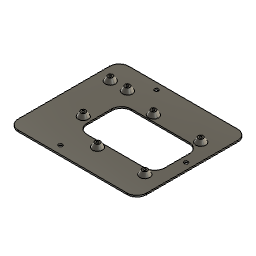
pi and feather sled (Autodesk Fusion 360 design; units mm, degrees)
Autodesk Fusion 360 part; units mm, degrees
sketch "Sketch1" plane through (0, 0, 0) normal (0, 0, 1) x (1, 0, 0)
  line L0 (0, 0) -> (203, 0) construction
  line L1 (203, 0) -> (203, 151) construction
  line L2 (203, 151) -> (0, 151) construction
  line L3 (0, 151) -> (0, 0) construction
  line L4 (101.5, 151) -> (101.5, 0) construction
  line L5 (0, 75.5) -> (203, 75.5) construction
  circle A0 centre (25.85, 110.5) radius 2
  circle A1 centre (61.05, 125.25) radius 2
  circle A2 centre (21, 75.5) radius 2
  circle A3 centre (101.5, 125.25) radius 2
  circle A4 centre (141.95, 125.25) radius 2
  circle A5 centre (177.15, 110.5) radius 2
  circle A6 centre (182, 75.5) radius 2
  circle A7 centre (25.85, 40.5) radius 2
  circle A8 centre (101.5, 25.75) radius 2
  circle A9 centre (61.05, 25.75) radius 2
  circle A10 centre (141.95, 25.75) radius 2
  circle A11 centre (177.15, 40.5) radius 2
  line L6 (122.4543, 101.192) -> (171.4543, 101.192) construction
  line L7 (171.4543, 101.192) -> (171.4543, 43.192) construction
  line L8 (171.4543, 43.192) -> (122.4543, 43.192) construction
  line L9 (122.4543, 43.192) -> (122.4543, 101.192) construction
  line L10 (118.9543, 124.692) -> (174.9543, 124.692) construction
  line L11 (174.9543, 124.692) -> (174.9543, 39.692) construction
  line L12 (174.9543, 39.692) -> (118.9543, 39.692) construction
  line L13 (118.9543, 39.692) -> (118.9543, 124.692) construction
  circle A12 centre (122.4543, 101.192) radius 1.15
  circle A13 centre (171.4543, 101.192) radius 1.15
  circle A14 centre (171.4543, 43.192) radius 1.15
  circle A15 centre (122.4543, 43.192) radius 1.15
  circle A16 centre (122.4543, 101.192) radius 2.65
  circle A17 centre (171.4543, 101.192) radius 2.65
  circle A18 centre (171.4543, 43.192) radius 2.65
  circle A19 centre (122.4543, 43.192) radius 2.65
  line L14 (55.9879, 132.0749) -> (188.973, 132.0749)
  line L15 (188.973, 132.0749) -> (188.973, 17.4198)
  line L16 (188.973, 17.4198) -> (55.9879, 17.4198)
  line L17 (55.9879, 17.4198) -> (55.9879, 132.0749)
  line L18 (69.6743, 109.192) -> (87.4543, 109.192) construction
  line L19 (87.4543, 109.192) -> (87.4543, 63.472) construction
  line L20 (87.4543, 63.472) -> (69.6743, 63.472) construction
  line L21 (69.6743, 63.472) -> (69.6743, 109.192) construction
  circle A20 centre (69.6743, 109.192) radius 1.15
  circle A21 centre (69.6743, 109.192) radius 2.65
  circle A22 centre (87.4543, 109.192) radius 2.65
  circle A23 centre (87.4543, 109.192) radius 1.15
  circle A24 centre (69.6743, 63.472) radius 2.65
  circle A25 centre (69.6743, 63.472) radius 1.15
  circle A26 centre (87.4543, 63.472) radius 2.65
  circle A27 centre (87.4543, 63.472) radius 1.15
  line L22 (95.4972, 94.9899) -> (175.7715, 94.9899)
  line L23 (175.7715, 94.9899) -> (175.7715, 49.2006)
  line L24 (175.7715, 49.2006) -> (95.4972, 49.2006)
  line L25 (95.4972, 49.2006) -> (95.4972, 94.9899)
  point P0 (61.05, 125.25)
  point P1 (25.85, 110.5)
  point P2 (177.15, 110.5)
  point P3 (141.95, 125.25)
  point P4 (177.15, 40.5)
  point P5 (141.95, 25.75)
  point P6 (61.05, 25.75)
  point P7 (25.85, 40.5)
  point P8 (101.5, 125.25)
  point P9 (21, 75.5)
  point P10 (182, 75.5)
  point P11 (101.5, 25.75)
  point P12 (61.05, 25.75)
  point P13 (141.95, 25.75)
  point P14 (177.15, 40.5)
  dimension "d1" = 203
  dimension "d2" = 151
  dimension "d3" = 161
  dimension "d4" = 151.3
  dimension "d5" = 80.9
  dimension "d6" = 70
  dimension "d7" = 99.5
  dimension "d8" = 99.5
  dimension "d10" = 4
  dimension "d12" = 4
  dimension "d14" = 4
  dimension "d16" = 4
  dimension "d19" = 49
  dimension "d20" = 58
  dimension "d21" = 56
  dimension "d22" = 85
  dimension "d23" = 3.5
  dimension "d24" = 3.5
  dimension "d25" = 2.3
  dimension "d26" = 2.3
  dimension "d27" = 2.3
  dimension "d28" = 2.3
  dimension "d29" = 1.5
  dimension "d30" = 1.5
  dimension "d31" = 1.5
  dimension "d32" = 1.5
  dimension "d41" = 45.72
  dimension "d42" = 17.78
  dimension "d43" = 2.3
  dimension "d44" = 1.5
  dimension "d47" = 17.78
  dimension "d48" = -45.72
  dimension "d54" = 35
  dimension "d55" = 8
  constraint horizontal L0
  constraint vertical L1
  constraint horizontal L2
  constraint vertical L3
  constraint coincident L0.start L3.end
  constraint midpoint L2 L4.start
  constraint midpoint L0 L4.end
  constraint midpoint L3 L5.start
  constraint midpoint L1 L5.end
  constraint symmetric L4 P0 P3
  constraint symmetric L4 P1 P2
  constraint symmetric L5 P0 P12
  constraint symmetric L5 P1 P7
  constraint symmetric L5 P2 P14
  constraint symmetric L5 P3 P13
  constraint coincident L4 P8
  constraint coincident L5 P9
  constraint symmetric L4 P9 P10
  constraint symmetric L5 P8 P11
  constraint coincident P1 A0.centre
  constraint coincident P0 A1.centre
  constraint coincident P8 A3.centre
  constraint symmetric L4 A0 A5
  constraint symmetric L4 A1 A4
  constraint symmetric L4 A2 A6
  constraint symmetric L5 A0 A7
  constraint symmetric L5 A3 A8
  constraint symmetric L5 A1 A9
  constraint symmetric L5 A4 A10
  constraint symmetric L5 A5 A11
  constraint coincident P9 A2.centre
  constraint horizontal L6
  constraint vertical L7
  constraint horizontal L8
  constraint vertical L9
  constraint horizontal L10
  constraint vertical L11
  constraint horizontal L12
  constraint vertical L13
  constraint coincident L6.start L9.end
  constraint coincident L6.end L7.start
  constraint coincident L7.end L8.start
  constraint coincident L8.end L9.start
  constraint concentric A12 A16
  constraint concentric A13 A17
  constraint concentric A14 A18
  constraint concentric A15 A19
  constraint horizontal L14
  constraint vertical L15
  constraint horizontal L16
  constraint vertical L17
  constraint horizontal L18
  constraint vertical L19
  constraint horizontal L20
  constraint vertical L21
  constraint coincident L18.start L21.end
  constraint concentric A20 A21
  constraint horizontal L22
  constraint vertical L23
  constraint horizontal L24
  constraint vertical L25
  measures "d1" distance of L0.start L0.end
  measures "d2" distance of L0.start L2.end
  measures "d3" distance of P9 P10
  measures "d4" distance of P1 P2
  measures "d5" distance of P0 P3
  measures "d6" distance of P1 P7
  measures "d7" distance of P0 P12
  measures "d8" distance of P8 P11
  measures "d10" diameter of A0
  measures "d12" diameter of A1
  measures "d14" diameter of A2
  measures "d16" diameter of A3
  measures "d19" distance of L6.start L6.end
  measures "d20" distance of L6.start L8.end
  measures "d21" distance of L10.start L10.end
  measures "d22" distance of L10.start L12.end
  measures "d23" distance of L8 L12
  measures "d24" distance of L9 L13
  measures "d25" diameter of A12
  measures "d26" diameter of A13
  measures "d27" diameter of A14
  measures "d28" diameter of A15
  measures "d29" distance of A12 A16
  measures "d30" distance of A15 A19
  measures "d31" distance of A13 A17
  measures "d32" distance of A14 A18
  measures "d41" distance of L18.start L20.end
  measures "d42" distance of L18.start L18.end
  measures "d43" diameter of A20
  measures "d44" distance of A20 A21
  measures "d54" horizontal distance of L8.end L19.end
  measures "d55" vertical distance of L6.start L18.end
extrude "Extrude2" add sketch "Sketch1" along normal blind 1.5 contours A1 | A4 | A5 | A9 | A10 | A11 | A16 | A17 | A18 | A19 | L14 L15 L16 L17 | A21 | A22 | A24 | A25 | A26
extrude "Extrude3" add sketch "Sketch1" along normal blind 6 contours A16 | A17 | A18 | A19 | A21 | A22 | A26
draft "Draft1" angle 30 neutral plane through (0, 0, 6) pull (0, 0, 1) 7 faces at (120.1931, 102.5738, 3) (171.5204, 103.8412, 3) (171.5204, 45.8412, 3) (125.0912, 43.4559, 3) (71.9356, 110.5738, 3) (89.7156, 110.5738, 3) (90.0912, 63.7359, 3)
fillet "Fillet1" radius 10 8 edges at (55.9879, 17.4198, 0.75) (188.973, 17.4198, 0.75) (188.973, 132.0749, 0.75) (55.9879, 132.0749, 0.75) (95.4972, 94.9899, 0.75) (95.4972, 49.2006, 0.75) (175.7715, 94.9899, 0.75) (175.7715, 49.2006, 0.75)
